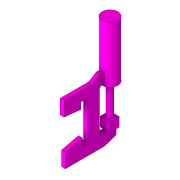
# Autodesk Inventor part: Sustitue Clamp
Saved by Autodesk Inventor 2020.1 (Build 241239000, 239)
## iProperties
Created: 2019-09-16
Part Number: Sustitue Clamp
Material: Generic
Document SubType Name: Modeling
Designer: thomastremblay
Density: 1 g/cm^3
Appearance: Magenta
Author: thomastremblay
Autodesk Inventor part; units mm, degrees
ref_plane "YZ Plane" through (0, 0, 0) normal (1, 0, 0) x (0, 1, 0)
ref_plane "XZ Plane" through (0, 0, 0) normal (0, 1, 0) x (-1, 0, 0)
ref_plane "XY Plane" through (0, 0, 0) normal (0, 0, 1) x (1, 0, 0)
sketch "Sketch1" plane through (0, 0, 0) normal (1, 0, 0) x (0, 0, -1)
  line L0 (76.417, -156.0446) -> (38.7716, -168.593)
  line L1 (38.7716, -168.593) -> (-87.6783, -168.593)
  line L2 (-87.6783, -168.593) -> (-87.6783, -123.2255)
  line L3 (-87.6783, -123.2255) -> (-32.6581, -109.7118)
  line L4 (-32.6581, -109.7118) -> (-32.6581, -129.9824)
  line L5 (-32.6581, -129.9824) -> (76.417, -129.9824)
  line L6 (76.417, -129.9824) -> (76.417, -156.0446)
  line L7 (-16.2486, -129.9824) -> (-16.2486, -7.8675)
  line L8 (-16.2486, -7.8675) -> (-37.4845, -7.8675)
  line L9 (-37.4845, -7.8675) -> (-37.4845, -28.1467)
  line L10 (-37.4845, -28.1467) -> (-91.5394, -22.8377)
  line L11 (-91.5394, -22.8377) -> (-91.5394, 23.4951)
  line L12 (-91.5394, 23.4951) -> (0, 23.4951)
  line L13 (0, 23.4951) -> (21.8795, 37.0088)
  arc A0 (38.3256, 14.8774) -> (21.8795, 37.0088) centre (29.1509, 25.2359) ccw
  line L14 (38.3256, 14.8774) -> (21.8883, 0.3187)
  line L15 (21.8883, 0.3187) -> (21.8795, -129.9824)
  line L16 (76.417, -129.9824) -> (76.417, -100.2282)
  line L17 (76.417, -100.2282) -> (46.4938, -100.2282)
  line L18 (46.4938, -100.2282) -> (46.4938, -129.9824)
  line L19 (46.4938, -129.9824) -> (76.417, -129.9824)
  point P0 (0, 0)
  constraints: 40 end point, 10 perpendicular, 2 parallel, 2 point on circle, 2 point on line, 2 tangent, 1 centre point, 1 midpoint
extrude "Extrusion1" add sketch "Sketch1" along normal mid plane 12.7 contours L0 L1 L2 L3 L4 L5 L6 | L5 L7 L8 L9 L10 L11 L12 L13 A0 L14 L15
extrude "Extrusion2" add sketch "Sketch1" along normal mid plane 31.75 contours L5 L18 L17 L16
sketch "Sketch2" plane through (15.875, -100.2282, -76.417) normal (0, 1, 0) x (-1, 0, 0)
  circle A0 centre (15.875, 13.936) radius 9.5136
  point P0 (15.875, 76.417)
  constraints: 1 centre point
extrude "Extrusion3" add sketch "Sketch2" along normal blind 98.425
sketch "Sketch3" plane through (0, -1.8032, -62.481) normal (0, 1, 0) x (1, 0, 0)
  circle A0 centre (0, 0) radius 25.4
  point P0 (0, -62.481)
  dimension "d6" = 50.8
  constraints: 1 centre point
  measures "d6" diameter of A0
extrude "Extrusion4" add sketch "Sketch3" along normal blind 180.34
sketch "Sketch4" plane through (6.35, 0, 0) normal (1, 0, 0) x (0, 0, -1)
  arc A0 (37.8876, 35.9665) -> (21.8795, 37.0088) centre (29.1509, 25.2359) ccw projected
  point P0 (0, 0)
  point P1 (22.8739, -26.7555)
  constraints: 1 coincident
hole "Hole1" at (6.35, 25.2359, -29.1509) direction (-1, 0, 0) diameter 12.7 end through all
body "Solid1"
